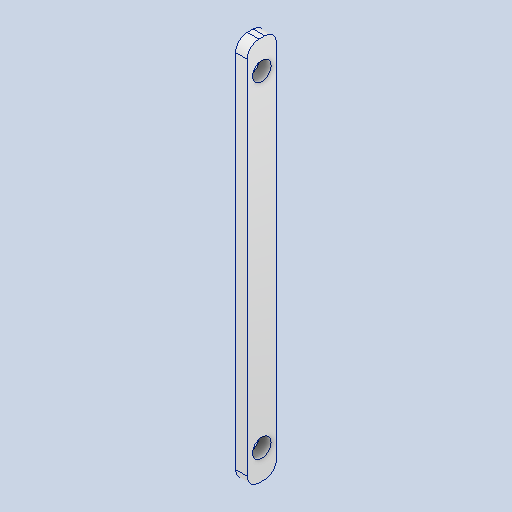
# Autodesk Inventor part: base_weel-v2-Plate-10
Saved by Autodesk Inventor 2025.2 (Build 292293000, 293)
## iProperties
Created: 2025-02-08
Part Number: base_weel-v2-Plate-10
Material: アルミニウム 6061
Document SubType Name: Modeling
Designer: haruy
Density: 2.7 g/cm^3
Appearance: アルミニウム - フラット
Author: haruy
Autodesk Inventor part; units mm, degrees
ref_plane "YZ Plane" through (0, 0, 0) normal (1, 0, 0) x (0, 1, 0)
ref_plane "XZ Plane" through (0, 0, 0) normal (0, 1, 0) x (-1, 0, 0)
ref_plane "XY Plane" through (0, 0, 0) normal (0, 0, 1) x (1, 0, 0)
derived "base_weel-v2-Plate-1.ipt"
sketch "スケッチ1" plane through (0, 0, 0) normal (1, 0, 0) x (0, 1, 0)
  line L0 (-315, 315) -> (315, 315)
  line L1 (315, 315) -> (315, -315)
  line L2 (315, -315) -> (-315, -315)
  line L3 (-315, -315) -> (-315, 315)
  line L4 (-315, 315) -> (315, -315) construction
  line L5 (315, 315) -> (-315, -315) construction
  line L6 (-295, 218) -> (-295, -202)
  line L7 (-295, -202) -> (-315, -202)
  line L8 (-315, -202) -> (-315, 210)
  line L9 (242, 315) -> (-242, 315)
  line L10 (-242, 315) -> (-242, 295)
  line L11 (-242, 295) -> (242, 295)
  line L12 (242, 295) -> (242, 315)
  line L13 (-295, 218) -> (-295, 315)
  line L14 (0, 0) -> (-956.5973, 0)
  circle A0 centre (0, 0) radius 400
  line L15 (-330, 25) -> (-380, 25)
  line L16 (-380, 25) -> (-380, -25)
  line L17 (-380, -25) -> (-330, -25)
  line L18 (-330, -25) -> (-330, 25)
  line L19 (0, 0) -> (0, -630.9179)
  line L20 (-315, 40) -> (-395, 40)
  line L21 (-395, 40) -> (-395, 30)
  line L22 (-395, 30) -> (-315, 30)
  line L23 (-315, 30) -> (-315, 40)
  line L24 (-395, 30) -> (-385, 30)
  line L25 (-385, 30) -> (-385, 0)
  line L26 (-385, 0) -> (-395, 0)
  line L27 (-395, 0) -> (-395, 30)
  line L28 (295, 202) -> (315, 202)
  line L29 (315, 202) -> (315, -202)
  line L30 (315, -202) -> (295, -202)
  line L31 (295, -202) -> (295, 202)
  line L32 (-222.2183, -315) -> (242, -315)
  line L33 (242, -315) -> (242, -295)
  line L34 (242, -295) -> (-242, -295)
  line L35 (315, 315) -> (0, 0) construction
  line L36 (315, 125) -> (315, 145)
  circle A1 centre (548.4769, 0) radius 122.5
  circle A2 centre (179.6905, 0) radius 600
  circle A3 centre (548.4769, 0) radius 200
  circle A4 centre (0, 0) radius 10 construction
  arc A5 (0, 150) -> (0, -150) centre (0, 0) ccw
  arc A6 (0, 140) -> (0, -140) centre (0, 0) ccw
  line L37 (-146.3272, 32.9904) -> (-136.572, 30.791)
  line L38 (-137.5812, 37.6817) -> (-140.4404, 25)
  line L39 (-140.4404, 25) -> (-145.318, 26.0997)
  line L40 (-145.318, 26.0997) -> (-142.4588, 38.7814)
  line L41 (-142.4588, 38.7814) -> (-137.5812, 37.6817)
  arc A7 (-29.1302, 142.0438) -> (-29.1302, -142.0438) centre (0, 0) ccw
  circle A8 centre (-151.4904, 39.2799) radius 6.5
  circle A9 centre (-129.0401, 34.2184) radius 6.5 construction
  circle A10 centre (-129.0401, 34.2184) radius 1.5 construction
  circle A11 centre (-151.4904, 39.2799) radius 1.5
  line L42 (-30.1668, 22.5) -> (-174.1362, 22.5) construction
  line L43 (-174.1362, 22.5) -> (-174.1362, 7.5)
  line L44 (-174.1362, 7.5) -> (-30.1668, 7.5) construction
  line L45 (-30.1668, 7.5) -> (-30.1668, 22.5) construction
  line L46 (-146.3272, -32.9904) -> (-136.572, -30.791)
  line L47 (-137.5812, -37.6817) -> (-140.4404, -25)
  line L48 (-140.4404, -25) -> (-145.318, -26.0997)
  line L49 (-145.318, -26.0997) -> (-142.4588, -38.7814)
  line L50 (-142.4588, -38.7814) -> (-137.5812, -37.6817)
  circle A12 centre (-151.4904, -39.2799) radius 6.5
  circle A13 centre (-129.0401, -34.2184) radius 6.5 construction
  circle A14 centre (-129.0401, -34.2184) radius 1.5 construction
  circle A15 centre (-151.4904, -39.2799) radius 1.5
  line L51 (-30.1668, -22.5) -> (-174.1362, -22.5) construction
  line L52 (-174.1362, -22.5) -> (-174.1362, -7.5)
  line L53 (-174.1362, -7.5) -> (-30.1668, -7.5) construction
  line L54 (-30.1668, -7.5) -> (-30.1668, -22.5) construction
  line L55 (-151.4904, 39.2799) -> (-129.0401, 34.2184) construction
  line L56 (-129.0401, 34.2184) -> (-129.59, 31.7796) construction
  line L57 (-129.59, 31.7796) -> (-152.0402, 36.8412) construction
  line L58 (-152.0402, 36.8412) -> (-151.4904, 39.2799) construction
  line L59 (-129.0401, 34.2184) -> (-151.4904, 39.2799) construction
  line L60 (-151.4904, 39.2799) -> (-150.9405, 41.7187) construction
  line L61 (-150.9405, 41.7187) -> (-128.4903, 36.6572) construction
  line L62 (-128.4903, 36.6572) -> (-129.0401, 34.2184) construction
  line L63 (-128.4903, 36.6572) -> (-129.59, 31.7796) construction
  line L64 (-129.59, 31.7796) -> (-117.8838, 29.1404) construction
  line L65 (-117.8838, 29.1404) -> (-116.7841, 34.0179) construction
  line L66 (-116.7841, 34.0179) -> (-128.4903, 36.6572) construction
  line L67 (-150.9405, 41.7187) -> (-152.0402, 36.8412) construction
  line L68 (-152.0402, 36.8412) -> (-163.7464, 39.4804) construction
  line L69 (-163.7464, 39.4804) -> (-162.6467, 44.358) construction
  line L70 (-162.6467, 44.358) -> (-150.9405, 41.7187) construction
  line L71 (-155.2683, 45.2572) -> (-128.9412, 39.3216)
  line L72 (-128.9412, 39.3216) -> (-132.2403, 24.6889)
  line L73 (-132.2403, 24.6889) -> (-158.5673, 30.6245)
  line L74 (-158.5673, 30.6245) -> (-155.2683, 45.2572)
  line L75 (-155.2683, -45.2572) -> (-128.9412, -39.3216)
  line L76 (-128.9412, -39.3216) -> (-132.2403, -24.6889)
  line L77 (-132.2403, -24.6889) -> (-158.5673, -30.6245)
  line L78 (-158.5673, -30.6245) -> (-155.2683, -45.2572)
  arc A16 (-132.2403, 24.6889) -> (-132.2403, -24.6889) centre (0, 0) ccw
  arc A17 (-158.5673, 30.6245) -> (-158.5673, -30.6245) centre (0, 0) ccw
  circle A18 centre (-152.5, 15) radius 1.25
  line L79 (-145, 0) -> (-145, 74.7382)
  circle A19 centre (-137.5, 15) radius 1.25
  circle A20 centre (-152.5, -15) radius 1.25
  circle A21 centre (-137.5, -15) radius 1.25
  line L80 (0, 0) -> (0, 140)
  line L81 (0, 0) -> (-47.8828, 131.557) construction
  line L82 (0, 140) -> (0, 150)
  line L83 (-137.5846, 25.8938) -> (-134.2855, 40.5265)
  line L84 (-137.5846, -25.8938) -> (-134.2855, -40.5265)
  circle A22 centre (0, 0) radius 20 construction
  line L85 (295, 45) -> (-295, 45)
  line L86 (-295, 45) -> (-295, 25)
  line L87 (-295, 25) -> (295, 25)
  line L88 (295, 25) -> (295, 45)
  line L89 (-40, 295) -> (-50, 295)
  line L90 (-50, 295) -> (-50, 45)
  line L91 (-50, 45) -> (-40, 45)
  line L92 (-40, 45) -> (-40, 295)
  line L93 (295, -45) -> (-295, -45)
  line L94 (-295, -25) -> (295, -25)
  line L95 (-50, -295) -> (-50, -45)
  line L96 (-40, -45) -> (-40, -295)
  line L97 (-40, 45) -> (-40, -45)
  line L98 (40, 45) -> (40, -45)
  circle A23 centre (20, 35) radius 1.5 construction
  circle A24 centre (-20, 35) radius 1.5 construction
  circle A25 centre (20, -35) radius 1.5 construction
  circle A26 centre (-20, -35) radius 1.5 construction
  circle A27 centre (-45, 125) radius 1.5
  circle A28 centre (-45, 125) radius 5
  circle A29 centre (-130, 35) radius 5
  circle A30 centre (-130, 35) radius 1.5
  line L99 (-40, 134.1641) -> (-40, 125)
  line L100 (-50, 125) -> (-50, 130.767)
  line L101 (-137.7498, 25) -> (-127.5801, 30.6246)
  line L102 (-132.5707, 45) -> (-126.366, 38.4342)
  circle A31 centre (-45, -125) radius 1.5
  circle A32 centre (-45, -125) radius 5
  circle A33 centre (-130, -35) radius 5
  circle A34 centre (-130, -35) radius 1.5
  line L103 (-40, -134.1641) -> (-40, -125)
  line L104 (-50, -125) -> (-50, -130.767)
  line L105 (-137.7498, -25) -> (-127.5801, -30.6246)
  line L106 (-132.5707, -45) -> (-126.366, -38.4342)
  circle A35 centre (0, 0) radius 18.6
  line L107 (-242, -295) -> (-242, -315)
  line L108 (242, 315) -> (222, 315)
  line L109 (222, 315) -> (222, 295)
  line L110 (222, 295) -> (242, 295)
  line L111 (242, 295) -> (242, 315)
  line L112 (242, -315) -> (222, -315)
  line L113 (222, -315) -> (222, -295)
  line L114 (222, -295) -> (242, -295)
  line L115 (242, -295) -> (242, -315)
  line L116 (197, 295) -> (295, 197)
  line L117 (295, 197) -> (284.3934, 186.3934)
  line L118 (284.3934, 186.3934) -> (186.3934, 284.3934)
  line L119 (186.3934, 284.3934) -> (197, 295)
  line L120 (197, 295) -> (197, 315)
  line L121 (197.9167, 294.0833) -> (187.3101, 283.4767)
  line L122 (198.2703, 272.5165) -> (272.5165, 198.2703)
  line L123 (272.5165, 198.2703) -> (231.5043, 157.2581)
  line L124 (231.5043, 157.2581) -> (157.2581, 231.5043)
  line L125 (157.2581, 231.5043) -> (198.2703, 272.5165)
  line L126 (290.9013, 201.0987) -> (280.2947, 190.4921)
  line L127 (93.7624, 295) -> (295, 93.7624)
  line L128 (295, 93.7624) -> (284.3934, 83.1558)
  line L129 (284.3934, 83.1558) -> (83.1558, 284.3934)
  line L130 (214.1802, 277.8198) -> (203.5736, 267.2132)
  line L131 (277.8198, 214.1802) -> (267.2132, 203.5736)
  circle A36 centre (199.6845, 281.7089) radius 1.5
  circle A37 centre (213.8266, 267.5668) radius 1.6
  line L132 (186.3934, 284.3934) -> (175.7868, 295)
  circle A38 centre (187, 305) radius 1.5
  circle A39 centre (177, 305) radius 1.5
  line L133 (172, 315) -> (172, 295)
  line L134 (93.7624, 295) -> (93.7624, 295)
  line L135 (93.7624, 295) -> (93.7624, 315)
  line L136 (83.1558, 284.3934) -> (72.5492, 295)
  line L137 (68.7624, 315) -> (68.7624, 295)
  line L138 (284.3934, 186.3934) -> (295, 175.7868)
  line L139 (295, 197) -> (315, 197)
  line L140 (295, 93.7624) -> (295, 93.7624)
  line L141 (284.3934, 83.1558) -> (295, 72.5492)
  line L142 (-197, 295) -> (-295, 197)
  line L143 (-284.3934, 186.3934) -> (-186.3934, 284.3934)
  line L144 (-197, 295) -> (-197, 315)
  line L145 (-197.9167, 294.0833) -> (-187.3101, 283.4767)
  line L146 (-272.5165, 198.2703) -> (-231.5043, 157.2581)
  line L147 (-157.2581, 231.5043) -> (-198.2703, 272.5165)
  line L148 (-290.9013, 201.0987) -> (-280.2947, 190.4921)
  line L149 (-93.7624, 295) -> (-295, 93.7624)
  line L150 (-295, 93.7624) -> (-284.3934, 83.1558)
  line L151 (-284.3934, 83.1558) -> (-83.1558, 284.3934)
  line L152 (-83.1558, 284.3934) -> (-93.7624, 295)
  line L153 (-214.1802, 277.8198) -> (-203.5736, 267.2132)
  line L154 (-186.3934, 284.3934) -> (-175.7868, 295)
  line L155 (-172, 315) -> (-172, 295)
  line L156 (-93.7624, 295) -> (-93.7624, 315)
  line L157 (-83.1558, 284.3934) -> (-72.5492, 295)
  line L158 (-68.7624, 315) -> (-68.7624, 295)
  line L159 (-284.3934, 186.3934) -> (-295, 175.7868)
  line L160 (-295, 197) -> (-315, 197)
  line L161 (-284.3934, 83.1558) -> (-295, 72.5492)
  line L162 (197, -295) -> (295, -197)
  line L163 (284.3934, -186.3934) -> (186.3934, -284.3934)
  line L164 (197.9167, -294.0833) -> (187.3101, -283.4767)
  line L165 (290.9013, -201.0987) -> (280.2947, -190.4921)
  line L166 (93.7624, -295) -> (295, -93.7624)
  line L167 (295, -93.7624) -> (284.3934, -83.1558)
  line L168 (284.3934, -83.1558) -> (83.1558, -284.3934)
  line L169 (83.1558, -284.3934) -> (93.7624, -295)
  line L170 (-93.7624, -295) -> (-295, -93.7624)
  line L171 (-83.1558, -284.3934) -> (-93.7624, -295)
  line L172 (-284.3934, -83.1558) -> (-83.1558, -284.3934)
  line L173 (-295, -93.7624) -> (-284.3934, -83.1558)
  line L174 (-284.3934, -186.3934) -> (-186.3934, -284.3934)
  line L175 (-197, -295) -> (-295, -197)
  line L176 (-197.9167, -294.0833) -> (-187.3101, -283.4767)
  line L177 (-214.1802, -277.8198) -> (-203.5736, -267.2132)
  line L178 (-290.9013, -201.0987) -> (-280.2947, -190.4921)
  line L179 (242, 295) -> (222, 295)
  arc A40 (0, 86) -> (0, -86) centre (0, 0) ccw
  circle A41 centre (-90.8667, 48.5) radius 21
  circle A42 centre (0, 0) radius 124
  circle A43 centre (-90.8667, 48.5) radius 17
  arc A44 (40.4951, 75.8693) -> (0, 86) centre (0, 0) ccw
  line L180 (-40, 45) -> (-50, 45)
  line L181 (-50, 45) -> (-50, -45)
  line L182 (-50, -45) -> (-40, -45)
  line L183 (-40, -45) -> (-40, 45)
  line L184 (-40, 295) -> (-50, 295)
  line L185 (-50, 295) -> (-50, 315)
  line L186 (-50, 315) -> (-40, 315)
  line L187 (-40, 315) -> (-40, 295)
  line L188 (-40, -295) -> (-50, -295)
  line L189 (-50, -295) -> (-50, -315)
  line L190 (-50, -315) -> (-40, -315)
  line L191 (-40, -315) -> (-40, -295)
  line L192 (50, 295) -> (50, 45)
  line L193 (40, 45) -> (40, 295)
  line L194 (50, -295) -> (50, -45)
  line L195 (40, -45) -> (40, -295)
  line L196 (50, 45) -> (50, -45)
  line L197 (40, -45) -> (40, 45)
  line L198 (50, 295) -> (50, 315)
  line L199 (40, 315) -> (40, 295)
  line L200 (50, -295) -> (50, -315)
  line L201 (40, -315) -> (40, -295)
  line L202 (-40.4092, 123.019) -> (-35, 135.5544)
  line L203 (-48.7417, 121.6834) -> (-55, 128.7439)
  line L204 (-40.4092, -123.019) -> (-35, -135.5544)
  line L205 (-48.7417, -121.6834) -> (-55, -128.7439)
  arc A45 (40.4951, 75.8693) -> (-40.4951, -75.8693) centre (0, 0) ccw
  circle A46 centre (0, 0) radius 86 construction
  circle A47 centre (0, 0) radius 78.5
  circle A48 centre (-45, 58) radius 1.5
  circle A49 centre (-45, 58) radius 5
  circle A50 centre (45, 58) radius 5
  circle A51 centre (45, 58) radius 1.5
  line L206 (46.5549, 53.2479) -> (55, 56.0112)
  line L207 (40.325, 56.2267) -> (35, 70.2656)
  line L208 (50, 60.5165) -> (50, 69.9714)
  arc A52 (50, 69.9714) -> (40.4951, 75.8693) centre (0, 0) ccw
  line L209 (-40.325, 56.2267) -> (-35, 70.2656)
  line L210 (-46.5549, 53.2479) -> (-55, 56.0112)
  circle A53 centre (-45, -58) radius 1.5
  circle A54 centre (-45, -58) radius 5
  line L211 (-40.325, -56.2267) -> (-35, -70.2656) construction
  line L212 (-46.5549, -53.2479) -> (-55, -56.0112)
  line L213 (-40, -67.5444) -> (-40, -76.1315)
  arc A55 (-40.526, -75.8528) -> (-40, -76.1315) centre (0, 0) ccw
  line L214 (-40, -76.1315) -> (-40, -58)
  line L215 (222.6655, 269.3345) -> (212.0589, 258.7279)
  line L216 (295, 197) -> (315, 197)
  line L217 (294.0833, 197.9167) -> (283.4767, 187.3101)
  circle A56 centre (281.7089, 199.6845) radius 1.5
  circle A57 centre (267.5668, 213.8266) radius 1.6
  circle A58 centre (305, 187) radius 1.5
  circle A59 centre (305, 177) radius 1.5
  line L218 (315, 172) -> (295, 172)
  line L219 (269.3345, 222.6655) -> (258.7279, 212.0589)
  circle A60 centre (83.7624, 305) radius 1.5
  circle A61 centre (73.7624, 305) radius 1.5
  line L220 (197.9167, 294.0833) -> (94.6791, 294.0833)
  line L221 (187.3101, 283.4767) -> (84.0725, 283.4767)
  line L222 (94.6791, 294.0833) -> (84.0725, 283.4767)
  circle A62 centre (96.4469, 281.7089) radius 1.5
  circle A63 centre (110.5891, 267.5668) radius 1.5
  line L223 (119.4279, 269.3345) -> (108.8213, 258.7279)
  line L224 (295, 93.7624) -> (315, 93.7624)
  line L225 (315, 68.7624) -> (295, 68.7624)
  circle A64 centre (305, 83.7624) radius 1.5
  circle A65 centre (305, 73.7624) radius 1.5
  line L226 (294.0833, 94.6791) -> (283.4767, 84.0725)
  circle A66 centre (281.7089, 96.4469) radius 1.5
  circle A67 centre (267.5668, 110.5891) radius 1.5
  line L227 (269.3345, 119.4279) -> (258.7279, 108.8213)
  line L228 (-197, 295) -> (-197, 315)
  line L229 (-197.9167, 294.0833) -> (-187.3101, 283.4767)
  line L230 (-214.1802, 277.8198) -> (-203.5736, 267.2132)
  circle A68 centre (-199.6845, 281.7089) radius 1.5
  circle A69 centre (-213.8266, 267.5668) radius 1.6
  circle A70 centre (-187, 305) radius 1.5
  circle A71 centre (-177, 305) radius 1.5
  line L231 (-172, 315) -> (-172, 295)
  line L232 (-93.7624, 295) -> (-93.7624, 315)
  line L233 (-68.7624, 315) -> (-68.7624, 295)
  line L234 (-295, 197) -> (-315, 197)
  line L235 (-222.6655, 269.3345) -> (-212.0589, 258.7279)
  line L236 (-269.3345, 222.6655) -> (-258.7279, 212.0589)
  circle A72 centre (-267.5668, 213.8266) radius 1.6
  circle A73 centre (-281.7089, 199.6845) radius 1.5
  line L237 (-294.0833, 197.9167) -> (-283.4767, 187.3101)
  line L238 (-315, 172) -> (-295, 172)
  circle A74 centre (-305, 177) radius 1.5
  circle A75 centre (-305, 187) radius 1.5
  circle A76 centre (-83.7624, 305) radius 1.5
  circle A77 centre (-73.7624, 305) radius 1.5
  line L239 (-94.6791, 294.0833) -> (-84.0725, 283.4767)
  circle A78 centre (-96.4469, 281.7089) radius 1.5
  circle A79 centre (-110.5891, 267.5668) radius 1.5
  line L240 (-119.4279, 269.3345) -> (-108.8213, 258.7279)
  line L241 (-295, 93.7624) -> (-315, 93.7624)
  line L242 (-315, 68.7624) -> (-295, 68.7624)
  circle A80 centre (-305, 73.7624) radius 1.5
  circle A81 centre (-305, 83.7624) radius 1.5
  line L243 (-294.0833, 94.6791) -> (-283.4767, 84.0725)
  circle A82 centre (-281.7089, 96.4469) radius 1.5
  circle A83 centre (-267.5668, 110.5891) radius 1.5
  line L244 (-269.3345, 119.4279) -> (-258.7279, 108.8213)
  line L245 (197, -295) -> (197, -315)
  line L246 (197.9167, -294.0833) -> (187.3101, -283.4767)
  circle A84 centre (199.6845, -281.7089) radius 1.5
  circle A85 centre (213.8266, -267.5668) radius 1.6
  circle A86 centre (187, -305) radius 1.5
  circle A87 centre (177, -305) radius 1.5
  line L247 (172, -315) -> (172, -295)
  line L248 (93.7624, -295) -> (93.7624, -315)
  line L249 (68.7624, -315) -> (68.7624, -295)
  line L250 (295, -197) -> (315, -197)
  line L251 (-197, -295) -> (-197, -315)
  line L252 (-172, -315) -> (-172, -295)
  line L253 (-68.7624, -315) -> (-68.7624, -295)
  line L254 (-197.9167, -294.0833) -> (-187.3101, -283.4767)
  line L255 (-295, -197) -> (-315, -197)
  line L256 (222.6655, -269.3345) -> (212.0589, -258.7279)
  line L257 (269.3345, -222.6655) -> (258.7279, -212.0589)
  circle A88 centre (267.5668, -213.8266) radius 1.6
  circle A89 centre (281.7089, -199.6845) radius 1.5
  line L258 (294.0833, -197.9167) -> (283.4767, -187.3101)
  line L259 (315, -172) -> (295, -172)
  circle A90 centre (305, -177) radius 1.5
  circle A91 centre (305, -187) radius 1.5
  circle A92 centre (83.7624, -305) radius 1.5
  circle A93 centre (73.7624, -305) radius 1.5
  line L260 (94.6791, -294.0833) -> (84.0725, -283.4767)
  circle A94 centre (96.4469, -281.7089) radius 1.5
  circle A95 centre (110.5891, -267.5668) radius 1.5
  line L261 (119.4279, -269.3345) -> (108.8213, -258.7279)
  line L262 (295, -93.7624) -> (315, -93.7624)
  line L263 (315, -68.7624) -> (295, -68.7624)
  circle A96 centre (305, -73.7624) radius 1.5
  circle A97 centre (305, -83.7624) radius 1.5
  line L264 (294.0833, -94.6791) -> (283.4767, -84.0725)
  circle A98 centre (281.7089, -96.4469) radius 1.5
  circle A99 centre (267.5668, -110.5891) radius 1.5
  line L265 (269.3345, -119.4279) -> (258.7279, -108.8213)
  circle A100 centre (-177, -305) radius 1.5
  circle A101 centre (-187, -305) radius 1.5
  circle A102 centre (-199.6845, -281.7089) radius 1.5
  circle A103 centre (-213.8266, -267.5668) radius 1.6
  line L266 (-222.6655, -269.3345) -> (-212.0589, -258.7279)
  circle A104 centre (-267.5668, -213.8266) radius 1.6
  line L267 (-269.3345, -222.6655) -> (-258.7279, -212.0589)
  circle A105 centre (-281.7089, -199.6845) radius 1.5
  line L268 (-294.0833, -197.9167) -> (-283.4767, -187.3101)
  circle A106 centre (-305, -187) radius 1.5
  circle A107 centre (-305, -177) radius 1.5
  line L269 (-315, -172) -> (-295, -172)
  line L270 (-295, -93.7624) -> (-315, -93.7624)
  line L271 (-315, -68.7624) -> (-295, -68.7624)
  circle A108 centre (-305, -73.7624) radius 1.5
  circle A109 centre (-305, -83.7624) radius 1.5
  line L272 (-294.0833, -94.6791) -> (-283.4767, -84.0725)
  circle A110 centre (-281.7089, -96.4469) radius 1.5
  circle A111 centre (-267.5668, -110.5891) radius 1.5
  line L273 (-269.3345, -119.4279) -> (-258.7279, -108.8213)
  line L274 (-119.4279, -269.3345) -> (-108.8213, -258.7279)
  circle A112 centre (-110.5891, -267.5668) radius 1.5
  circle A113 centre (-96.4469, -281.7089) radius 1.5
  line L275 (-94.6791, -294.0833) -> (-84.0725, -283.4767)
  line L276 (-93.7624, -295) -> (-93.7624, -315)
  circle A114 centre (-73.7624, -305) radius 1.5
  circle A115 centre (-83.7624, -305) radius 1.5
  line L277 (-295, 202) -> (-315, 202)
  line L278 (265, 45) -> (265, 25)
  circle A116 centre (275, 35) radius 1.5
  circle A117 centre (285, 35) radius 1.5
  circle A118 centre (305, 35) radius 1.5
  circle A119 centre (305, 25) radius 1.5
  line L279 (295, 25) -> (315, 25)
  line L280 (265, -45) -> (265, -25)
  circle A120 centre (275, -35) radius 1.5
  circle A121 centre (285, -35) radius 1.5
  circle A122 centre (305, -35) radius 1.5
  circle A123 centre (305, -25) radius 1.5
  line L281 (-265, 45) -> (-265, 25)
  circle A124 centre (-275, 35) radius 1.5
  circle A125 centre (-285, 35) radius 1.5
  circle A126 centre (-305, 35) radius 1.5
  circle A127 centre (-305, 25) radius 1.5
  line L282 (-265, -45) -> (-265, -25)
  circle A128 centre (-275, -35) radius 1.5
  circle A129 centre (-285, -35) radius 1.5
  circle A130 centre (-305, -35) radius 1.5
  circle A131 centre (-305, -25) radius 1.5
  circle A132 centre (48, 345) radius 44
  circle A133 centre (-50, 345) radius 44
  circle A134 centre (-50, 345) radius 15
  line L283 (295, 45) -> (315, 45)
  line L284 (295, 15) -> (315, 15)
  line L285 (-315, 45.5) -> (-390, 45.5)
  line L286 (-390, 45.5) -> (-390, 0)
  line L287 (-390, 0) -> (-315, 0)
  line L288 (-315, 0) -> (-315, 45.5)
  circle A135 centre (-305, 48) radius 1.5
  circle A136 centre (-305, -48) radius 1.5
  line L289 (114.7878, 210) -> (54.7878, 210)
  line L290 (54.7878, 210) -> (54.7878, 270)
  line L291 (54.7878, 270) -> (114.7878, 270)
  line L292 (114.7878, 270) -> (114.7878, 210)
  line L293 (34.7878, 210) -> (-25.2122, 210)
  line L294 (-25.2122, 210) -> (-25.2122, 270)
  line L295 (-25.2122, 270) -> (34.7878, 270)
  line L296 (34.7878, 270) -> (34.7878, 210)
  line L297 (-45.2122, 250) -> (-115.2122, 250)
  line L298 (-115.2122, 250) -> (-115.2122, 266)
  line L299 (-115.2122, 266) -> (-45.2122, 266)
  line L300 (-45.2122, 266) -> (-45.2122, 250)
  line L301 (-50.2122, 214) -> (-110.2122, 214)
  line L302 (-110.2122, 214) -> (-110.2122, 230)
  line L303 (-110.2122, 230) -> (-50.2122, 230)
  line L304 (-50.2122, 230) -> (-50.2122, 214)
  circle A137 centre (0, 0) radius 175.5
  line L305 (-185, -89) -> (-302, -89)
  line L306 (-302, -89) -> (-302, 89)
  line L307 (-302, 89) -> (-185, 89)
  line L308 (-185, 89) -> (-185, -89)
  line L309 (287, -17.7878) -> (205, -17.7878)
  line L310 (205, -17.7878) -> (205, 79.2122)
  line L311 (205, 79.2122) -> (287, 79.2122)
  line L312 (287, 79.2122) -> (287, -17.7878)
  line L313 (284.5, -114.7878) -> (207.5, -114.7878)
  line L314 (207.5, -114.7878) -> (207.5, -37.7878)
  line L315 (207.5, -37.7878) -> (284.5, -37.7878)
  line L316 (284.5, -37.7878) -> (284.5, -114.7878)
  line L317 (281, 99.2122) -> (211, 99.2122)
  line L318 (211, 99.2122) -> (211, 115.2122)
  line L319 (211, 115.2122) -> (281, 115.2122)
  line L320 (281, 115.2122) -> (281, 99.2122)
  line L321 (137.7122, 315) -> (-137.7122, 315)
  line L322 (-137.7122, 315) -> (-137.7122, 185)
  line L323 (-137.7122, 185) -> (137.7122, 185)
  line L324 (137.7122, 185) -> (137.7122, 315)
  line L325 (315, -137.7122) -> (185, -137.7122)
  line L326 (185, -137.7122) -> (185, 137.7122)
  line L327 (185, 137.7122) -> (315, 137.7122)
  line L328 (315, 137.7122) -> (315, -137.7122)
  line L329 (258.7782, 137.7122) -> (278.7782, 137.7122)
  line L330 (278.7782, 137.7122) -> (278.7782, 127.7122)
  line L331 (278.7782, 127.7122) -> (258.7782, 127.7122)
  line L332 (258.7782, 127.7122) -> (258.7782, 137.7122)
  circle A138 centre (268.7782, 132.7122) radius 1.5
  line L333 (278.7782, 137.7122) -> (231.1981, 137.7122)
  line L334 (231.1981, 137.7122) -> (231.1981, 147.7122)
  line L335 (231.1981, 147.7122) -> (278.7782, 147.7122)
  line L336 (278.7782, 147.7122) -> (278.7782, 137.7122)
  line L337 (255.1924, 112.3568) -> (233.9792, 133.57)
  line L338 (233.9792, 133.57) -> (230.4437, 130.0345)
  line L339 (230.4437, 130.0345) -> (251.6569, 108.8213)
  line L340 (251.6569, 108.8213) -> (255.1924, 112.3568)
  line L341 (288.78, 89.3758) -> (114.1246, 264.0312)
  line L342 (244.5858, 144.1766) -> (248.1213, 147.7122)
  line L343 (248.1213, 147.7122) -> (269.3345, 126.499)
  line L344 (269.3345, 126.499) -> (265.799, 122.9634)
  circle A139 centre (268.7782, 132.7122) radius 4
  line L345 (233.9792, 133.57) -> (244.5858, 144.1766)
  line L346 (-330, 143.5) -> (-340, 143.5)
  line L347 (-340, 143.5) -> (-340, -143.5)
  line L348 (-340, -143.5) -> (-330, -143.5)
  line L349 (-330, -143.5) -> (-330, 143.5)
  line L350 (-315, 119) -> (-295, 119)
  line L351 (-295, 119) -> (-295, 104)
  line L352 (-295, 104) -> (-315, 104)
  line L353 (-315, 104) -> (-315, 119)
  line L354 (-315, 153.5) -> (-325, 153.5)
  line L355 (-325, 153.5) -> (-325, 0)
  line L356 (-325, 0) -> (-315, 0)
  line L357 (-315, 0) -> (-315, 153.5)
  line L358 (-340, 133.5) -> (-345, 133.5)
  line L359 (-345, 133.5) -> (-345, 143.5)
  line L360 (-345, 143.5) -> (-340, 143.5)
  line L361 (-340, 143.5) -> (-340, 133.5)
  line L362 (-330, 133.5) -> (-325, 133.5)
  line L363 (-325, 133.5) -> (-325, 143.5)
  line L364 (-325, 143.5) -> (-330, 143.5)
  line L365 (-330, 143.5) -> (-330, 133.5)
  line L366 (-325, 153.5) -> (-345, 153.5)
  line L367 (-345, 153.5) -> (-345, 143.5)
  line L368 (-345, 143.5) -> (-325, 143.5)
  line L369 (-325, 143.5) -> (-325, 153.5)
  line L370 (-295, 104) -> (-345, 104)
  line L371 (-345, 104) -> (-345, 98)
  line L372 (-345, 98) -> (-295, 98)
  line L373 (-295, 98) -> (-295, 104)
  line L374 (185, -25) -> (180, -25)
  line L375 (180, -25) -> (180, -15)
  line L376 (180, -15) -> (185, -15)
  line L377 (185, -15) -> (185, -25)
  line L378 (185, -25) -> (195, -25)
  line L379 (195, -25) -> (195, -15)
  line L380 (195, -15) -> (185, -15)
  line L381 (185, -15) -> (185, -25)
  line L382 (40, 180) -> (30, 180)
  line L383 (30, 180) -> (30, 195)
  line L384 (30, 195) -> (40, 195)
  line L385 (40, 195) -> (40, 180)
  circle A140 centre (-132.7122, 268.7782) radius 1.5
  circle A141 centre (132.7122, 268.7782) radius 1.5
  line L386 (-243.5, 89) -> (-243.5, -89)
  circle A142 centre (-214, 35) radius 1.5
  circle A143 centre (-214, -35) radius 1.5
  line L387 (-214, 89) -> (-214, -89)
  line L388 (-246, 89) -> (-246, -89)
  circle A144 centre (-254.5, 35) radius 4
  circle A145 centre (-254.5, -35) radius 4
  circle A146 centre (0, 0) radius 100
  circle A147 centre (-134.1671, -14.9726) radius 5
  circle A148 centre (-134.1671, -14.9726) radius 1.25
  circle A149 centre (-134.9074, -5) radius 5
  circle A150 centre (-134.9074, -5) radius 1.25
  circle A151 centre (20, 35) radius 1.6
  circle A152 centre (-20, 35) radius 1.6
  circle A153 centre (-20, -35) radius 1.6
  circle A154 centre (20, -35) radius 1.6
  circle A155 centre (0, 0) radius 20 construction
  circle A156 centre (0, 0) radius 16 construction
  line L389 (-33, 21) -> (0, 21)
  line L390 (0, 21) -> (0, 16)
  line L391 (0, 16) -> (-33, 16)
  line L392 (-33, 16) -> (-33, 21)
  circle A157 centre (-28, 18.5) radius 1.6
  circle A158 centre (0, 0) radius 24 construction
  circle A159 centre (0, 0) radius 28 construction
  circle A160 centre (-28, 18.5) radius 4
  line L393 (33, 21) -> (0, 21)
  line L394 (0, 16) -> (33, 16)
  circle A161 centre (28, 18.5) radius 1.6
  line L395 (33, 16) -> (33, 21)
  line L396 (33, -21) -> (0, -21)
  line L397 (0, -16) -> (33, -16)
  line L398 (33, -16) -> (33, -21)
  circle A162 centre (28, -18.5) radius 1.6
  line L399 (-33, -21) -> (0, -21)
  line L400 (0, -16) -> (-33, -16)
  line L401 (-33, -16) -> (-33, -21)
  circle A163 centre (-28, -18.5) radius 1.6
  line L402 (252.0104, 177.7642) -> (177.7642, 252.0104)
  point P0 (-141.4496, 31.8907)
  point P1 (-129.0401, 34.2184)
  point P2 (-150, 0)
  point P3 (-242, 305)
  point P4 (-295, 93.7624)
  point P5 (-161.4975, 0)
  point P6 (305, 25)
  point P7 (295, 35)
extrude "押し出し1" add sketch "スケッチ1" along normal blind 2 contours L399 L401 L400 A35 L19 | L19 A35 L397 L398 L396 | A35 L400 L19 | L19 L397 A35
fillet "フィレット1" radius 2 4 edges at (1, -33, -16) (1, -33, -21) (1, 33, -21) (1, 33, -16)
